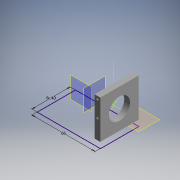
# Autodesk Inventor part: C-head-base
Saved by Autodesk Inventor 2016 (Build 200138000, 138)
## iProperties
Created: 2015-05-08
Part Number: C-head-base
Material: Generic
Document SubType Name: Modeling
Designer: ax
Density: 1 g/cm^3
Appearance: Default
Mass: 14.277 g
Surface Area: 72.4987 cm^2
Volume: 14.277 cm^3
cMotorSize: 40,000 mm
d1: 40,000 mm
d4: 6,000 mm
d5: 40,000 mm
d6: 40,000 mm
d7: 0,00 deg
d13: 20,000 mm
d16: 32,000 mm
d32: 22,000 mm
Author: ax
Autodesk Inventor part; units mm, degrees
ref_plane "YZ Plane" through (0, 0, 0) normal (1, 0, 0) x (0, 1, 0)
ref_plane "XZ Plane" through (0, 0, 0) normal (0, 1, 0) x (-1, 0, 0)
ref_plane "XY Plane" through (0, 0, 0) normal (0, 0, 1) x (1, 0, 0)
ref_plane "Work Plane3" through (0, 0, 6) normal (0, 0, 1) x (1, 0, 0)
sketch "Sketch2" plane through (0, 0, 6) normal (0, 0, 1) x (1, 0, 0)
  line L0 (0, 0) -> (-6, 0)
  line L1 (-6, 0) -> (-6, -40)
  line L2 (-6, -40) -> (0, -40)
  line L3 (0, -40) -> (0, 0)
  dimension "d4" = 6
  dimension "d5" = 40
  constraints: 8 end point, 2 parallel, 1 perpendicular
  measures "d4" distance of L2.end L1.end
  measures "d5" distance of L1.end L0.end
extrude "Extrusion2" add sketch "Sketch2" along normal blind 40
ref_plane "Work Plane4" through (-60, 0, 0) normal (0, 1, 0) x (1, 0, 0)
sketch "Sketch3" plane through (-60, 0, 0) normal (0, 1, 0) x (1, 0, 0)
  point P0 (60, 0)
ref_plane "Work Plane5" through (-6, -40, 46) normal (-1, 0, 0) x (0, 0, 1)
sketch "Sketch5" plane through (-6, -40, 46) normal (-1, 0, 0) x (0, 0, 1)
  line L0 (0, 20) -> (-20, 20)
  line L1 (0, 20) -> (20, 20) construction
  line L2 (-36, 36) -> (-4, 36)
  line L3 (-4, 36) -> (-4, 4)
  line L4 (-4, 4) -> (-36, 4)
  line L5 (-36, 4) -> (-36, 36)
  line L6 (-36, 36) -> (-4, 4) construction
  line L7 (-4, 36) -> (-36, 4) construction
  dimension "d13" = 20
  dimension "d14" = 180
  dimension "d16" = 32
  constraints: 16 end point, 2 coincident, 2 horizontal, 2 midpoint, 2 parallel, 2 perpendicular, 1 collinear
  measures "d13" distance of L0.start L0.end
  measures "d14" angle of L0 L1
  measures "d16" distance of L2.end L3.end
hole "Hole2" at (-6, -20, 26) direction (1, 0, 0) diameter 22 end through all
sketch "Sketch6" plane through (-6, -40, 6) normal (0, -1, 0) x (1, 0, 0)
  line L0 (0, 0) -> (6, 0) projected
  line L1 (6, 0) -> (6, 40) projected
  point P0 (3, 37)
  point P1 (3, 20)
  dimension "d47" = 37
  dimension "d48" = 20
  dimension "d49" = 3
  dimension "d50" = 3
  measures "d47" distance from line of L0 point (3, 37)
  measures "d48" distance from line of L0 point (3, 20)
  measures "d49" distance from line of L1 point (3, 20)
  measures "d50" distance from line of L1 point (3, 37)
hole "Hole3" at (-3, -40, 26) at (-3, -40, 43) direction (0, 1, 0) diameter 2.459 depth 8.8 tip angle 118 thread size "M3x0.5" class "6H" standard "ISO Metric profile"
sketch "Sketch7" plane through (-6, -40, 6) normal (0, -1, 0) x (1, 0, 0)
  point P0 (3, 20)
  point P1 (3, 37)
sketch "Sketch8" plane through (0, 0, 6) normal (0, 0, -1) x (-1, 0, 0)
  point P0 (3, -23)
  point P1 (3, -37)
hole "Hole5" at (-3, -23, 6) at (-3, -37, 6) direction (0, 0, 1) diameter 2.459 depth 7 tip angle 120 thread size "M3x0.5" class "6H" standard "ISO Metric profile"
equation "\"d5\" = d1"
equation "\"d6\" = cMotorSize"
equation "\"d13\" = 0.5 * cMotorSize"
equation "\"d48\" = 0.5 * cMotorSize"
equation "\"d50\" = d49"
equation "\"d1\" = cMotorSize"
equation "\"cMotorSize\" = 40"
body "Solid1"
